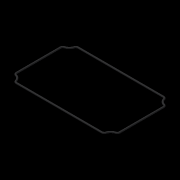
# Autodesk Inventor part: 3d_DAA - Glass o-ring 60x1
Saved by Autodesk Inventor 2018 (Build 220112000, 112)
## iProperties
Created: 2024-09-05
Part Number: 3d_DAA - Glass o-ring 60x1
Material: Goma NBR
Document SubType Name: Modeling
Designer: cda1
Density: 0.93 g/cm^3
Appearance: Goma - Negro
Author: cda1
Autodesk Inventor part; units mm, degrees
ref_plane "YZ Plane" through (0, 0, 0) normal (1, 0, 0) x (0, 1, 0)
ref_plane "XZ Plane" through (0, 0, 0) normal (0, 1, 0) x (-1, 0, 0)
ref_plane "XY Plane" through (0, 0, 0) normal (0, 0, 1) x (1, 0, 0)
sketch "Boceto1" plane through (0, 0, 0) normal (0, 0, 1) x (1, 0, 0)
  arc A0 (-31.034783, 14.617936) -> (-27.617936, 18.034783) centre (-32.3, 19.3) ccw construction
  arc A1 (-26.749099, 18.7) -> (-27.617936, 18.034783) centre (-26.749099, 17.8) ccw construction
  line L0 (26.749099, 18.7) -> (-26.749099, 18.7) construction
  arc A2 (27.617936, 18.034783) -> (26.749099, 18.7) centre (26.749099, 17.8) ccw construction
  arc A3 (27.617936, 18.034783) -> (31.034783, 14.617936) centre (32.3, 19.3) ccw construction
  arc A4 (31.7, 13.749099) -> (31.034783, 14.617936) centre (30.8, 13.749099) ccw construction
  line L1 (31.7, -13.749099) -> (31.7, 13.749099) construction
  arc A5 (31.034783, -14.617936) -> (31.7, -13.749099) centre (30.8, -13.749099) ccw construction
  arc A6 (31.034783, -14.617936) -> (27.617936, -18.034783) centre (32.3, -19.3) ccw construction
  arc A7 (26.749099, -18.7) -> (27.617936, -18.034783) centre (26.749099, -17.8) ccw construction
  line L2 (-26.749099, -18.7) -> (26.749099, -18.7) construction
  arc A8 (-27.617936, -18.034783) -> (-26.749099, -18.7) centre (-26.749099, -17.8) ccw construction
  arc A9 (-27.617936, -18.034783) -> (-31.034783, -14.617936) centre (-32.3, -19.3) ccw construction
  arc A10 (-31.7, -13.749099) -> (-31.034783, -14.617936) centre (-30.8, -13.749099) ccw construction
  line L3 (-31.7, 13.749099) -> (-31.7, -13.749099) construction
  arc A11 (-31.034783, 14.617936) -> (-31.7, 13.749099) centre (-30.8, 13.749099) ccw construction
  arc A12 (-26.749099, 19.9) -> (-28.776385, 18.347826) centre (-26.749099, 17.8) ccw construction
  arc A13 (-31.347826, 15.776385) -> (-28.776385, 18.347826) centre (-32.3, 19.3) ccw construction
  arc A14 (-31.347826, 15.776385) -> (-32.9, 13.749099) centre (-30.8, 13.749099) ccw construction
  line L4 (-32.9, -13.749099) -> (-32.9, 13.749099) construction
  arc A15 (-32.9, -13.749099) -> (-31.347826, -15.776385) centre (-30.8, -13.749099) ccw construction
  arc A16 (-28.776385, -18.347826) -> (-31.347826, -15.776385) centre (-32.3, -19.3) ccw construction
  arc A17 (-28.776385, -18.347826) -> (-26.749099, -19.9) centre (-26.749099, -17.8) ccw construction
  line L5 (26.749099, -19.9) -> (-26.749099, -19.9) construction
  arc A18 (26.749099, -19.9) -> (28.776385, -18.347826) centre (26.749099, -17.8) ccw construction
  arc A19 (31.347826, -15.776385) -> (28.776385, -18.347826) centre (32.3, -19.3) ccw construction
  arc A20 (31.347826, -15.776385) -> (32.9, -13.749099) centre (30.8, -13.749099) ccw construction
  line L6 (32.9, 13.749099) -> (32.9, -13.749099) construction
  arc A21 (32.9, 13.749099) -> (31.347826, 15.776385) centre (30.8, 13.749099) ccw construction
  arc A22 (28.776385, 18.347826) -> (31.347826, 15.776385) centre (32.3, 19.3) ccw construction
  arc A23 (28.776385, 18.347826) -> (26.749099, 19.9) centre (26.749099, 17.8) ccw construction
  line L7 (-26.749099, 19.9) -> (26.749099, 19.9) construction
  arc A24 (28.19716, 18.191304) -> (26.749099, 19.3) centre (26.749099, 17.8) ccw
  arc A25 (28.19716, 18.191304) -> (31.191304, 15.19716) centre (32.3, 19.3) ccw
  arc A26 (32.3, 13.749099) -> (31.191304, 15.19716) centre (30.8, 13.749099) ccw
  line L8 (32.3, 13.749099) -> (32.3, -13.749099)
  arc A27 (31.191304, -15.19716) -> (32.3, -13.749099) centre (30.8, -13.749099) ccw
  arc A28 (31.191304, -15.19716) -> (28.19716, -18.191304) centre (32.3, -19.3) ccw
  arc A29 (26.749099, -19.3) -> (28.19716, -18.191304) centre (26.749099, -17.8) ccw
  line L9 (26.749099, -19.3) -> (-26.749099, -19.3)
  arc A30 (-28.19716, -18.191304) -> (-26.749099, -19.3) centre (-26.749099, -17.8) ccw
  arc A31 (-28.19716, -18.191304) -> (-31.191304, -15.19716) centre (-32.3, -19.3) ccw
  arc A32 (-32.3, -13.749099) -> (-31.191304, -15.19716) centre (-30.8, -13.749099) ccw
  line L10 (-32.3, -13.749099) -> (-32.3, 13.749099)
  arc A33 (-31.191304, 15.19716) -> (-32.3, 13.749099) centre (-30.8, 13.749099) ccw
  arc A34 (-31.191304, 15.19716) -> (-28.19716, 18.191304) centre (-32.3, 19.3) ccw
  arc A35 (-26.749099, 19.3) -> (-28.19716, 18.191304) centre (-26.749099, 17.8) ccw
  line L11 (-26.749099, 19.3) -> (26.749099, 19.3)
  point P0 (0, 0)
  dimension "d0" = 0.6
  constraints: 24 point on circle, 12 centre point, 8 end point, 15 other
  measures "d0" distance between parallel lines of L7 L11
sketch "Boceto2" plane through (0, 0, 0) normal (1, 0, 0) x (0, 1, 0)
  circle A0 centre (19.3, 0) radius 0.5
  point P0 (0, 0)
  point P1 (19.3, 0)
  dimension "d1" = 1
  constraints: 1 centre point, 1 coincident
  measures "d1" diameter of A0
sweep "Barrido1" add profiles "Boceto2" path "Boceto1"
